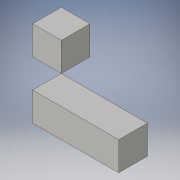
# Autodesk Inventor part: IED7_Sun_PuzzleCubeYellow
Saved by Autodesk Inventor 2016 (Build 200138000, 138)
## iProperties
Created: 2017-09-27
Part Number: IED7_Sun_PuzzleCubeYellow
Material: Generic
Document SubType Name: Sheet Metal
Designer: sun01147
Density: 1 g/cm^3
Sheet Metal Rule: Default
Appearance: Default
Author: sun01147
Autodesk Inventor part; units mm, degrees
ref_plane "YZ Plane" through (0, 0, 0) normal (1, 0, 0) x (0, 1, 0)
ref_plane "XZ Plane" through (0, 0, 0) normal (0, 1, 0) x (-1, 0, 0)
ref_plane "XY Plane" through (0, 0, 0) normal (0, 0, 1) x (1, 0, 0)
sketch "Sketch1" plane through (0, 0, 0) normal (0, 0, 1) x (1, 0, 0)
  line L0 (0, 57.15) -> (0, 0)
  line L1 (0, 57.15) -> (19.05, 57.15)
  line L2 (19.05, 57.15) -> (19.05, 19.05)
  line L3 (19.05, 19.05) -> (57.15, 19.05)
  line L4 (57.15, 19.05) -> (57.15, 0)
  line L5 (57.15, 0) -> (0, 0)
  line L6 (19.05, 19.05) -> (0, 19.05)
  line L7 (0, 19.05) -> (0, 38.1)
  line L8 (0, 38.1) -> (19.05, 38.1)
  dimension "d0" = 57.15
  dimension "d1" = 19.05
  dimension "d2" = 38.1
  dimension "d3" = 38.1
  dimension "d4" = 19.05
  constraints: 18 end point, 3 vertical, 2 horizontal, 2 perpendicular, 2 point on line, 1 midpoint
  measures "d0" distance of L0.start L0.end
  measures "d1" distance of L0.start L1.end
  measures "d2" distance of L1.end L2.end
  measures "d3" distance of L2.end L3.end
  measures "d4" distance of L7.end L8.end
extrude "Extrusion1" add sketch "Sketch1" against normal blind 19.05 contours L1 L2 L8 L0 | L6 L3 L4 L5 L0
equation "\"BendRadius\" = Thickness"
equation "\"BendReliefWidth\" = Thickness"
equation "\"BendReliefDepth\" = 0.5 * Thickness"
equation "\"CornerReliefSize\" = 4 * Thickness"
equation "\"MinimumRemnant\" = 2 * Thickness"
equation "\"TransitionRadius\" = BendRadius"
equation "\"JacobiRadiusSize\" = BendRadius"
equation "\"GapSize\" = Thickness"
equation "\"Thickness\" = 3.048"
body "Solid1"
